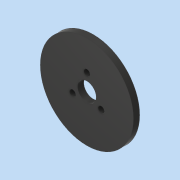
# Autodesk Inventor part: pistonSpurGear
Saved by Autodesk Inventor 2017 (Build 210142000, 142)
## iProperties
Created: 2016-11-28
Part Number: pistonSpurGear
Material: ABS Plastic
Document SubType Name: Modeling
Designer: techn
Density: 1.06 g/cm^3
Appearance: Smooth - Black
Author: techn
Autodesk Inventor part; units mm, degrees
ref_plane "YZ Plane" through (0, 0, 0) normal (1, 0, 0) x (0, 1, 0)
ref_plane "XZ Plane" through (0, 0, 0) normal (0, 1, 0) x (-1, 0, 0)
ref_plane "XY Plane" through (0, 0, 0) normal (0, 0, 1) x (1, 0, 0)
sketch "Sketch1" plane through (0, 0, 0) normal (0, 0, 1) x (1, 0, 0)
  circle A0 centre (0, 0) radius 23.495
  dimension "d0" = 46.99
  constraints: 1 centre point, 1 coincident
  measures "d0" diameter of A0
extrude "Extrusion1" add sketch "Sketch1" along normal blind 3.175
sketch "Sketch2" plane through (0, 0, 0) normal (0, 0, -1) x (-1, 0, 0)
  line L0 (0, 0) -> (0, 8.3295)
  circle A0 centre (0, 8.3295) radius 1.5875
  circle A1 centre (-7.2136, -4.1648) radius 1.5875
  circle A2 centre (7.2136, -4.1648) radius 1.5875
  dimension "d3" = 3.175
  dimension "d6" = 360
  dimension "d8" = 14.4272
  constraints: 3 centre point, 2 end point, 1 coincident, 1 vertical, 7 other
  measures "d3" diameter of A0
  measures "d8" distance of A2.centre L0.end
extrude "Extrusion2" cut sketch "Sketch2" against normal blind 3.175
sketch "Sketch3" plane through (0, 0, 3.175) normal (0, 0, 1) x (1, 0, 0)
  circle A0 centre (0, 0) radius 4.7625
  dimension "d11" = 9.525
  constraints: 1 centre point, 1 coincident
  measures "d11" diameter of A0
extrude "Extrusion3" cut sketch "Sketch3" against normal blind 3.175
body "Solid1"
